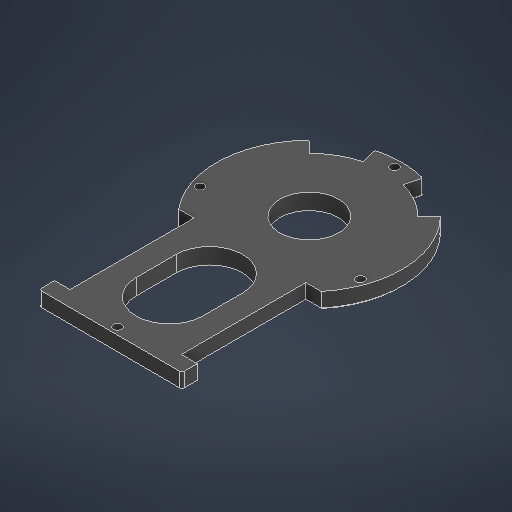
# Autodesk Inventor part: Tapa de caja reductora - eje z
Saved by Autodesk Inventor 2026 (Build 300175050, 175E)
## iProperties
Created: 2025-07-24
Part Number: Tapa de caja reductora - eje z
Material: Plastico PETG
Document SubType Name: Modeling
Designer: bello
Density: 1.27 g/cm^3
Appearance: Genérico
Author: bello
Autodesk Inventor part; units mm, degrees
ref_plane "YZ Plane" through (0, 0, 0) normal (1, 0, 0) x (0, 1, 0)
ref_plane "XZ Plane" through (0, 0, 0) normal (0, 1, 0) x (-1, 0, 0)
ref_plane "XY Plane" through (0, 0, 0) normal (0, 0, 1) x (1, 0, 0)
sketch "Boceto1" plane through (0, 0, 0) normal (0, 1, 0) x (-1, 0, 0)
  line L0 (26.7996, 74.6) -> (26.8, 68.8)
  line L1 (21, 68.8) -> (21, 22.2711)
  line L2 (7.5058, -28.0118) -> (9.0069, -33.6142)
  line L3 (-9.0069, -33.6142) -> (-7.5058, -28.0118)
  line L4 (-7.5058, -28.0118) -> (-9.0069, -33.6142)
  line L5 (-20.5061, -20.5061) -> (-24.6073, -24.6073)
  line L6 (-20.5061, -20.5061) -> (-24.6073, -24.6073)
  circle A0 centre (0, 0) radius 11
  line L7 (-21, 69) -> (-21, 22.2711)
  line L8 (-21, 22.2711) -> (-21, 69)
  line L9 (-26.7402, 22.2711) -> (-21, 22.2711)
  line L10 (-27, 74.8) -> (26.7996, 74.6)
  arc A1 (-9.0069, -33.6142) -> (9.0069, -33.6142) centre (0, 0) ccw
  arc A2 (-26.7402, 22.2711) -> (-24.6073, -24.6073) centre (0, 0) ccw
  arc A3 (24.6073, -24.6073) -> (26.7402, 22.2711) centre (0, 0) ccw
  line L11 (26.8, 68.8) -> (21, 68.8)
  line L12 (21, 22.2711) -> (26.7402, 22.2711)
  line L13 (-27, 74.8) -> (-27, 69)
  line L14 (-27, 69) -> (-21, 69)
  line L15 (24.6073, -24.6073) -> (20.3647, -20.3647)
  line L16 (7.5058, -28.0118) -> (7.454, -27.8187)
  line L17 (-7.5058, -28.0118) -> (-7.454, -27.8187)
  line L18 (-20.5061, -20.5061) -> (-20.3647, -20.3647)
  arc A4 (-20.3647, -20.3647) -> (-7.454, -27.8187) centre (0, 0) ccw
  arc A5 (7.454, -27.8187) -> (20.3647, -20.3647) centre (0, 0) ccw
  point P0 (0, 0)
  point P1 (0, 0)
  dimension "d3" = 53.8
  dimension "d5" = 22
  dimension "d15" = 5.8
  dimension "d16" = 46.5289
  constraints: 38 end point, 10 point on circle, 6 centre point, 3 collinear, 3 perpendicular, 3 point on line, 1 coincident, 1 horizontal, 1 vertical, 1 other
  measures "d3" distance of L10.start L0.start
  measures "d5" diameter of A0
  measures "d15" distance of L0.start L0.end
  measures "d16" distance of L1.start L1.end
extrude "Extrusión1" add sketch "Boceto1" along normal blind 6
fillet "Empalme2" radius 1 2 edges at (27, 3, 74.8) (-26.7996, 3, 74.6)
chamfer "Chaflán1" distance 0.6 angle 45 6 edges at (27, 0, 71.3981) (26.7058, 0, 74.5047) (0.0964, 0, 74.7) (-26.5081, 0, 74.3095) (-26.7998, 0, 71.2019) (24, 0, 69)
chamfer "Chaflán2" distance 0.6 angle 45 1 edges at (21, 0, 45.6355)
chamfer "Chaflán3" distance 0.6 angle 45 1 edges at (-21, 0, 45.5355)
chamfer "Chaflán4" distance 0.6 angle 45 2 edges at (-23.6, 0, 68.8) (-23.8701, 0, 22.2711)
chamfer "Chaflán5" distance 0.6 angle 45 3 edges at (-34.7443, 0, -1.9681) (-24.1144, 0, 21.6711) (-22.486, 0, -22.486)
chamfer "Chaflán6" distance 0.6 angle 45 9 edges at (-14.4, 0, -24.9415) (-8.2563, 0, -30.813) (0, 0, -34.8) (8.2563, 0, -30.813) (14.4, 0, -24.9415) (22.5567, 0, -22.5567) (34.764, 0, -1.5817) (23.8701, 0, 22.2711) (20.4, 0, 45.6355)
fillet "Empalme4" radius 0.5 4 edges at (-9.0069, 3.2998, -33.6142) (-24.6073, 3.2998, -24.6073) (9.0069, 3.2998, -33.6142) (24.6073, 3.2998, -24.6073)
sketch "Boceto2" plane through (0, 0, 0) normal (0, -1, 0) x (1, 0, 0)
  line L0 (0, 52.5) -> (0, 37.5) construction
  line L1 (-12.5, 52.5) -> (-12.5, 37.5)
  line L2 (12.5, 37.5) -> (12.5, 52.5)
  arc A0 (12.5, 52.5) -> (-12.5, 52.5) centre (0, 52.5) ccw
  arc A1 (-12.5, 37.5) -> (12.5, 37.5) centre (0, 37.5) ccw
  point P0 (0, 0)
  point P1 (0, 45)
  dimension "d43" = 25
  dimension "d44" = 15
  dimension "d45" = 37.5
  constraints: 8 end point, 4 point on circle, 4 tangent, 2 centre point, 1 midpoint, 1 parallel, 1 vertical
  measures "d43" diameter of A1
  measures "d44" distance of L0.end L0.start
  measures "d45" distance of point (0, 0) L0.end
extrude "Extrusión2" cut sketch "Boceto2" against normal blind 6
sketch "Boceto3" plane through (0, 6, 0) normal (0, 1, 0) x (1, 0, 0)
  circle A0 centre (0.0066, -72) radius 1.6
  circle A1 centre (0, 0) radius 32
  circle A2 centre (0, 32) radius 1.6
  circle A3 centre (-30.0702, -10.9446) radius 1.6
  circle A4 centre (30.0702, -10.9446) radius 1.6
  line L0 (0, 0) -> (-30.0702, -10.9446)
  line L1 (0, 0) -> (30.0702, -10.9446)
  line L2 (9.4586, 0) -> (-7.7353, 0)
  dimension "d48" = 64
  dimension "d49" = 3.2
  dimension "d50" = 20
  dimension "d51" = 20
  dimension "d53" = 72
  constraints: 6 end point, 5 centre point, 3 equal radius, 3 point on circle, 1 coincident, 1 horizontal
  measures "d48" diameter of A1
  measures "d49" diameter of A3
  measures "d50" angle of L2 L0
  measures "d51" angle of L2 L1
  measures "d53" vertical distance of A0.centre L2.end
extrude "Extrusión3" cut sketch "Boceto3" against normal through all contours A0 | A2 A1 | A1 A2 | A4 A1 | A1 L1 A4 | A1 A4 L1 | A3 L0 A1 | A1 A3 | L0 A3 A1
